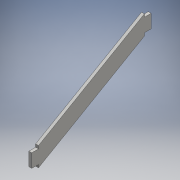
# Autodesk Inventor part: handle
Saved by Autodesk Inventor 2016 (Build 200138000, 138)
## iProperties
Created: 2015-09-14
Part Number: handle
Material: Generic
Document SubType Name: Modeling
Designer: Hulbert Office
Density: 1 g/cm^3
Appearance: Default
Author: Hulbert Office
Autodesk Inventor part; units mm, degrees
ref_plane "YZ Plane" through (0, 0, 0) normal (1, 0, 0) x (0, 1, 0)
ref_plane "XZ Plane" through (0, 0, 0) normal (0, 1, 0) x (-1, 0, 0)
ref_plane "XY Plane" through (0, 0, 0) normal (0, 0, 1) x (1, 0, 0)
sketch "Sketch2" plane through (0, 0, 0) normal (1, 0, 0) x (0, 1, 0)
  line L0 (0, -20) -> (80, -20) construction
  line L1 (0, -20) -> (110, 43.5085)
  line L2 (0, -20) -> (127.0171, -20) construction
  line L3 (110, 63.5085) -> (0, 0)
  line L4 (0, 0) -> (0, -3)
  line L5 (0, -3) -> (-7, -3)
  line L6 (-7, -3) -> (-7, -17)
  line L7 (-7, -17) -> (0, -17)
  line L8 (0, -17) -> (0, -20)
  line L9 (110, 63.5085) -> (110, 60.5085)
  line L10 (110, 60.5085) -> (117, 60.5085)
  line L11 (117, 60.5085) -> (117, 46.5085)
  line L12 (117, 46.5085) -> (110, 46.5085)
  line L13 (110, 46.5085) -> (110, 43.5085)
  line L14 (0, -3) -> (-5.1, -3)
  line L15 (0, -17) -> (-4, -17)
  dimension "d0" = 20
  dimension "d5" = 30
  dimension "d6" = 20
  dimension "d7" = 3
  dimension "d8" = 7
  dimension "d9" = 14
  dimension "d10" = 3
  dimension "d11" = 7
  dimension "d12" = 14
  dimension "d13" = 5.1
  dimension "d15" = 4
  constraints: 32 end point, 5 perpendicular, 3 point on line, 3 vertical, 2 horizontal, 1 equal length
  measures "d0" distance of L3.end L0.start
  measures "d5" angle of L2 L1
  measures "d6" distance of L1.end L3.start
  measures "d7" distance of L3.end L4.end
  measures "d8" distance of L4.end L5.end
  measures "d9" distance of L5.end L6.end
  measures "d10" distance of L3.start L9.end
  measures "d11" distance of L9.end L10.end
  measures "d12" distance of L10.end L11.end
  measures "d13" distance of L4.end L14.end
  measures "d15" distance of L7.end L15.end
extrude "Extrusion1" add sketch "Sketch2" along normal blind 3
body "Solid1"
